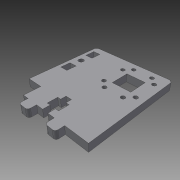
# Autodesk Inventor part: x_motor_cable_mount
Saved by Autodesk Inventor 2014 (Build 180170000, 170)
## iProperties
Created: 2013-12-02
Part Number: x_motor_cable_mount
Material: Generic
Document SubType Name: Modeling
Designer: buben
Density: 1 g/cm^3
Appearance: Default
Author: buben
Subject: Laser Cutted
Autodesk Inventor part; units mm, degrees
ref_plane "YZ Plane" through (0, 0, 0) normal (1, 0, 0) x (0, 1, 0)
ref_plane "XZ Plane" through (0, 0, 0) normal (0, 1, 0) x (-1, 0, 0)
ref_plane "XY Plane" through (0, 0, 0) normal (0, 0, 1) x (1, 0, 0)
sketch "Sketch1" plane through (0, 0, 0) normal (0, 0, 1) x (1, 0, 0)
  line L0 (12, 0) -> (64, 0)
  line L1 (64, 0) -> (64, 71.9)
  line L2 (64, 71.9) -> (0, 71.9)
  line L3 (0, 71.9) -> (0, 12)
  line L4 (3, 65.9) -> (9, 65.9)
  line L5 (9, 65.9) -> (9, 57.9)
  line L6 (9, 57.9) -> (3, 57.9)
  line L7 (3, 57.9) -> (3, 65.9)
  line L8 (3, 42.9) -> (9, 42.9)
  line L9 (9, 42.9) -> (9, 34.9)
  line L10 (9, 34.9) -> (3, 34.9)
  line L11 (3, 34.9) -> (3, 42.9)
  line L12 (0, 12) -> (12, 12)
  line L13 (12, 12) -> (12, 0)
  line L14 (3, 57.9) -> (9, 42.9) construction
  line L15 (3, 42.9) -> (9, 57.9) construction
  circle A0 centre (6, 50.4) radius 2.25
  point P0 (0, 0)
  dimension "d1" = 6
  dimension "d2" = 8
  dimension "d3" = 8
  dimension "d4" = 15
  dimension "d5" = 3
  dimension "d6" = 71.9
  dimension "d7" = 4.5
  dimension "d8" = 64
  dimension "d9" = 12
  dimension "d10" = 52
  dimension "d11" = 6
  constraints: 32 end point, 6 parallel, 5 perpendicular, 3 horizontal, 2 collinear, 1 centre point, 1 horizontal alignment, 1 midpoint, 1 vertical alignment
  measures "d1" distance of L4.start L4.end
  measures "d2" distance of L4.end L5.end
  measures "d3" distance of L8.end L9.end
  measures "d4" distance between parallel lines of L6 L8
  measures "d5" distance between parallel lines of L3 L7
  measures "d6" distance between parallel lines of L0 L2
  measures "d7" diameter of A0
  measures "d8" distance between parallel lines of L1 L3
  measures "d9" distance of L12.end L0.start
  measures "d10" distance of L0.start L0.end
  measures "d11" distance between parallel lines of L2 L4
extrude "Extrusion1" add sketch "Sketch1" along normal blind 6
sketch "Sketch2" plane through (0, 0, 6) normal (0, 0, 1) x (1, 0, 0)
  line L0 (64, 0) -> (64, 71.9) projected
  line L1 (12, 0) -> (64, 0) projected
  line L2 (29.75, 16.3) -> (34.25, 16.3)
  line L3 (34.25, 0) -> (29.75, 0)
  line L4 (36.75, 12.3) -> (36.75, 5)
  line L5 (27.25, 5) -> (27.25, 12.3)
  line L6 (29.75, 0) -> (29.75, 5)
  line L7 (29.75, 12.3) -> (29.75, 16.3)
  line L8 (27.25, 12.3) -> (29.75, 12.3)
  line L9 (34.25, 12.3) -> (36.75, 12.3)
  line L10 (34.25, 16.3) -> (34.25, 12.3)
  line L11 (34.25, 5) -> (34.25, 0)
  line L12 (36.75, 5) -> (34.25, 5)
  line L13 (29.75, 5) -> (27.25, 5)
  point P0 (0, 0)
  point P1 (32, 16.3)
  dimension "d14" = 2.5
  dimension "d15" = 2.5
  dimension "d16" = 4.5
  dimension "d17" = 5
  dimension "d18" = 7.3
  dimension "d19" = 4
  dimension "d20" = 32
  constraints: 24 end point, 10 parallel, 5 collinear, 4 perpendicular, 3 horizontal, 1 midpoint
  measures "d14" distance of L5.end L7.start
  measures "d15" distance of L9.start L4.start
  measures "d16" distance of L2.start L2.end
  measures "d17" distance of L11.start L3.start
  measures "d18" distance of L4.start L4.end
  measures "d19" distance of L2.end L9.start
  measures "d20" distance from line of L0 point (32, 16.3)
extrude "Extrusion2" cut sketch "Sketch2" against normal blind 6
sketch "Sketch3" plane through (0, 0, 6) normal (0, 0, 1) x (1, 0, 0)
  line L0 (34.25, 0) -> (64, 0) projected
  line L1 (12, 0) -> (29.75, 0) projected
  line L2 (29.75, 16.3) -> (34.25, 16.3) projected
  line L3 (16.5, 0) -> (24.5, 0)
  line L4 (24.5, 0) -> (24.5, -4)
  line L5 (22.5, -6) -> (18.5, -6)
  line L6 (16.5, -4) -> (16.5, 0)
  line L7 (39.5, 0) -> (47.5, 0)
  line L8 (47.5, 0) -> (47.5, -4)
  line L9 (45.5, -6) -> (41.5, -6)
  line L10 (39.5, -4) -> (39.5, 0)
  arc A0 (16.5, -4) -> (18.5, -6) centre (18.5, -4) ccw
  arc A1 (22.5, -6) -> (24.5, -4) centre (22.5, -4) ccw
  arc A2 (39.5, -4) -> (41.5, -6) centre (41.5, -4) ccw
  arc A3 (45.5, -6) -> (47.5, -4) centre (45.5, -4) ccw
  point P0 (0, 0)
  point P1 (32, 16.3)
  dimension "d23" = 2
  dimension "d24" = 8
  dimension "d25" = 8
  dimension "d26" = 6
  dimension "d27" = 15
  dimension "d28" = 7.5
  constraints: 16 end point, 8 point on circle, 8 tangent, 4 centre point, 4 parallel, 3 equal radius, 2 horizontal, 2 perpendicular, 2 point on line, 1 collinear, 1 midpoint
  measures "d23" radius of A0
  measures "d24" distance between parallel lines of L4 L6
  measures "d25" distance between parallel lines of L8 L10
  measures "d26" distance between parallel lines of L1 L5
  measures "d27" distance between parallel lines of L10 L4
  measures "d28" distance from line of point (32, 16.3) L4
extrude "Extrusion3" add sketch "Sketch3" against normal blind 6
chamfer "Chamfer1" distance 2 angle 45 2 edges at (0, 71.9, 3) (64, 71.9, 3)
sketch "Sketch4" plane through (0, 0, 0) normal (0, 0, -1) x (-1, 0, 0)
  line L0 (-64, 69.9) -> (-64, 0) projected
  line L1 (-2, 71.9) -> (-62, 71.9) projected
  line L2 (-39, 58.9) -> (-53, 58.9)
  line L3 (-53, 58.9) -> (-53, 44.9)
  line L4 (-53, 44.9) -> (-39, 44.9)
  line L5 (-39, 44.9) -> (-39, 58.9)
  line L6 (-34, 65.9) -> (-58, 65.9) construction
  line L7 (-58, 65.9) -> (-58, 37.9) construction
  line L8 (-58, 37.9) -> (-34, 37.9) construction
  line L9 (-34, 37.9) -> (-34, 65.9) construction
  circle A0 centre (-58, 60.9) radius 1.6
  circle A1 centre (-58, 42.9) radius 1.6
  circle A2 centre (-53, 37.9) radius 1.6
  circle A3 centre (-39, 37.9) radius 1.6
  circle A4 centre (-34, 42.9) radius 1.6
  circle A5 centre (-34, 60.9) radius 1.6
  circle A6 centre (-39, 65.9) radius 1.6
  circle A7 centre (-53, 65.9) radius 1.6
  point P0 (0, 0)
  point P1 (-58, 51.9)
  point P2 (-53, 51.9)
  point P3 (-46, 37.9)
  point P4 (-46, 44.9)
  dimension "d34" = 3.2
  dimension "d35" = 5
  dimension "d36" = 5
  dimension "d37" = 5
  dimension "d38" = 5
  dimension "d39" = 5
  dimension "d40" = 5
  dimension "d41" = 5
  dimension "d42" = 5
  dimension "d43" = 14
  dimension "d44" = 14
  dimension "d45" = 5
  dimension "d46" = 7
  dimension "d47" = 6
  dimension "d48" = 6
  constraints: 16 end point, 8 centre point, 8 point on line, 7 equal radius, 4 midpoint, 4 parallel, 2 horizontal, 2 perpendicular, 1 horizontal alignment, 1 vertical alignment
  measures "d34" diameter of A0
  measures "d35" distance of L6.end A0.centre
  measures "d36" distance of L7.end A1.centre
  measures "d37" distance of A2.centre L7.end
  measures "d38" distance of L8.end A3.centre
  measures "d39" distance of A4.centre L8.end
  measures "d40" distance of L6.start A5.centre
  measures "d41" distance of L6.start A6.centre
  measures "d42" distance of L6.end A7.centre
  measures "d43" distance of L2.start L2.end
  measures "d44" distance of L2.end L3.end
  measures "d45" distance between parallel lines of L9 L5
  measures "d46" distance between parallel lines of L6 L2
  measures "d47" distance between parallel lines of L1 L6
  measures "d48" distance between parallel lines of L0 L7
extrude "Extrusion4" cut sketch "Sketch4" against normal through all
equation "\"d36\" = d35"
equation "\"d37\" = d35"
equation "\"d38\" = d35"
equation "\"d39\" = d35"
equation "\"d40\" = d35"
equation "\"d41\" = d35"
equation "\"d42\" = d35"
body "Solid1"
